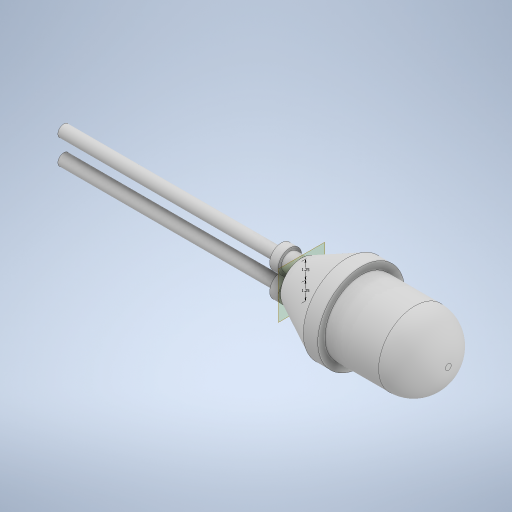
# Autodesk Inventor part: АЛ307
Saved by Autodesk Inventor 2024 (Build 280153000, 153)
## iProperties
Created: 2023-12-14
Part Number: АЛ307
Material: Generic
Document SubType Name: Sheet Metal
Designer: user
Density: 1 g/cm^3
Sheet Metal Rule: Default
Appearance: Default
Author: user
Autodesk Inventor part; units mm, degrees
ref_plane "YZ Plane" through (0, 0, 0) normal (1, 0, 0) x (0, 1, 0)
ref_plane "XZ Plane" through (0, 0, 0) normal (0, 1, 0) x (-1, 0, 0)
ref_plane "XY Plane" through (0, 0, 0) normal (0, 0, 1) x (1, 0, 0)
sketch "Sketch1" plane through (0, 0, 0) normal (0, 0, 1) x (1, 0, 0)
  line L0 (9.5185, 2.5022) -> (7.5185, 2.5022)
  line L1 (13.514, 0) -> (13.514, 0.2022)
  line L2 (11.214, 2.5022) -> (9.5185, 2.5022)
  arc A0 (13.514, 0.2022) -> (11.214, 2.5022) centre (11.214, 0.2022) ccw
  line L3 (13.514, 0) -> (3.514, 0)
  line L4 (-13, 1.25) -> (2, 1.25)
  line L5 (2, 1.65) -> (2.6, 1.65)
  line L6 (2.6, 1.65) -> (2.6, 1.45)
  line L7 (2.6, 1.45) -> (3.4, 1.45)
  line L8 (3.4, 1.45) -> (6.5185, 3)
  line L9 (-13, 1.25) -> (-13, 0.45)
  line L10 (-13, 0.45) -> (2, 0.45)
  line L11 (2, 0.45) -> (2, 0.05)
  line L12 (2, 0.05) -> (2.6, 0.05)
  line L13 (2.6, 0.05) -> (2.6, 0.25)
  line L14 (2.6, 0.25) -> (3.4, 0.25)
  line L15 (3.4, 1.45) -> (3.4, 0.25)
  line L16 (2, 1.65) -> (2, 1.25)
  line L17 (7.5185, 2.5022) -> (9.5185, 2.5022)
  arc A1 (3.514, 0) -> (3.4, 0.25) centre (3.1152, -0.0309) ccw
  line L18 (6.5185, 0) -> (6.5185, 0)
  line L19 (6.5185, 0) -> (6.5185, 3)
  line L20 (6.5185, 3) -> (7.5185, 3)
  line L21 (7.5185, 3) -> (7.5185, 0)
  dimension "d8" = 3
  dimension "d13" = 2.3
  dimension "d14" = 10
  dimension "d17" = 15
  dimension "d23" = 0.6
  dimension "d24" = 0.2
  dimension "d25" = 0.8
  dimension "d26" = 0.8
  dimension "d27" = 15
  dimension "d28" = 0.4
  dimension "d29" = 0.6
  dimension "d30" = 0.2
  dimension "d31" = 2
  dimension "d32" = 0.4
  dimension "d33" = 3
  dimension "d34" = 1
  constraints: 45 end point, 6 perpendicular, 6 vertical, 4 point on circle, 3 horizontal, 2 centre point, 2 point on line, 2 tangent, 1 collinear
  measures "d8" distance of L8.end L18.start
  measures "d13" radius of A0
  measures "d14" distance of L3.end L1.start
  measures "d17" distance of L4.start L4.end
  measures "d23" distance of L5.start L5.end
  measures "d24" distance of L5.end L6.end
  measures "d25" distance of L6.end L7.end
  measures "d26" distance of L4.start L9.end
  measures "d27" distance of L9.end L10.end
  measures "d28" distance of L10.end L11.end
  measures "d29" distance of L11.end L12.end
  measures "d30" distance of L12.end L13.end
  measures "d31" distance of L0.end L0.start
  measures "d32" radius of A1
  measures "d33" distance of L18.end L8.end
  measures "d34" distance of L8.end L20.end
revolve "Revolution1" add sketch "Sketch1" angle 360 about axis through (13.514, 0, 0) along (-1, 0, 0) contours L2 A0 L1 L3 L21 L0 | L21 L3 L19 L20 | L19 L3 A1 L15 L8
ref_plane "Work Plane1" through (3.4, 0, 0) normal (-1, 0, 0) x (0, 0, 1)
sketch "Sketch2" plane through (3.4, 0, 0) normal (-1, 0, 0) x (0, 0, 1)
  point P0 (0, 0)
sketch "Sketch3" plane through (3.4, 0, 0) normal (-1, 0, 0) x (0, 0, 1)
  line L0 (0, 0) -> (0, -1.25)
  line L1 (0, 0) -> (0, 1.25)
  dimension "d39" = 1.25
  dimension "d40" = 1.25
  constraints: 4 end point, 2 vertical
  measures "d39" distance of L0.start L0.end
  measures "d40" distance of L0.start L1.end
sketch "Sketch4" plane through (0, 0, 0) normal (0, 0, 1) x (1, 0, 0)
  line L0 (3.4021, -1.4575) -> (2.6021, -1.4575)
  line L1 (2.6021, -1.4575) -> (2.6021, -1.6575)
  line L2 (2.6021, -1.6575) -> (2.0021, -1.6575)
  line L3 (2.0021, -1.6575) -> (2.0021, -1.2575)
  line L4 (2.0021, -1.2575) -> (-12.9979, -1.2575)
  line L5 (-12.9979, -1.2575) -> (-12.9979, -0.4575)
  line L6 (-12.9979, -0.4575) -> (2.0021, -0.4575)
  line L7 (2.0021, -0.4575) -> (2.0021, -0.0575)
  line L8 (2.0021, -0.0575) -> (2.6021, -0.0575)
  line L9 (2.6021, -0.0575) -> (2.6021, -0.2575)
  line L10 (2.6021, -0.2575) -> (3.4021, -0.2575)
  line L11 (3.4021, -0.2575) -> (3.4021, -1.4575)
  line L12 (-12.9979, -0.8575) -> (3.4021, -0.8575)
  point P0 (0, 0)
  dimension "d41" = 0.8
  dimension "d42" = 0.2
  dimension "d43" = 0.6
  dimension "d44" = 0.4
  dimension "d45" = 15
  dimension "d46" = 0.8
  dimension "d47" = 15
  dimension "d48" = 0.4
  dimension "d49" = 0.6
  dimension "d50" = 0.2
  dimension "d51" = 0.8
  constraints: 26 end point, 7 perpendicular, 2 midpoint, 2 point on line, 1 horizontal, 1 vertical
  measures "d41" distance of L0.start L0.end
  measures "d42" distance of L0.end L1.end
  measures "d43" distance of L1.end L2.end
  measures "d44" distance of L2.end L3.end
  measures "d45" distance of L3.end L4.end
  measures "d46" distance of L4.end L5.end
  measures "d47" distance of L5.end L6.end
  measures "d48" distance of L6.end L7.end
  measures "d49" distance of L7.end L8.end
  measures "d50" distance of L8.end L9.end
  measures "d51" distance of L9.end L10.end
revolve "Revolution2" add sketch "Sketch4" angle 360 about axis through (-12.9979, -0.8575, 0) along (1, 0, 0) contours L0 L1 L2 L3 L4 L5 L12 L11
mirror "Mirror1" about plane through (0, 0, 0) normal (0, 1, 0) of "Revolution2"
equation "\"BendRadius\" = Thickness"
equation "\"BendReliefWidth\" = Thickness"
equation "\"BendReliefDepth\" = 0.5 * Thickness"
equation "\"CornerReliefSize\" = 4 * Thickness"
equation "\"MinimumRemnant\" = 2 * Thickness"
equation "\"TransitionRadius\" = BendRadius"
equation "\"JacobiRadiusSize\" = BendRadius"
equation "\"GapSize\" = Thickness"
equation "\"Thickness\" = 3.048"
body "Solid1"
